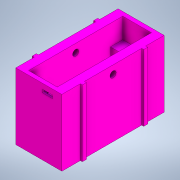
# Autodesk Inventor part: hull_servo
Saved by Autodesk Inventor 2020 (Build 240168000, 168)
## iProperties
Created: 2019-09-18
Part Number: hull_servo
Material: Generic
Document SubType Name: Modeling
Designer: suchanek
Density: 1 g/cm^3
Appearance: Default
Author: suchanek
Autodesk Inventor part; units mm, degrees
ref_plane "YZ Plane" through (0, 0, 0) normal (1, 0, 0) x (0, 1, 0)
ref_plane "XZ Plane" through (0, 0, 0) normal (0, 1, 0) x (-1, 0, 0)
ref_plane "XY Plane" through (0, 0, 0) normal (0, 0, 1) x (1, 0, 0)
sketch "Sketch1" plane through (0, 0, 0) normal (0, 1, 0) x (-1, 0, 0)
  line L0 (-14, 34) -> (14, 34)
  line L1 (14, 34) -> (14, -34)
  line L2 (14, -34) -> (-14, -34)
  line L3 (-14, -34) -> (-14, 34)
  line L4 (-14, 34) -> (14, -34) construction
  line L5 (14, 34) -> (-14, -34) construction
  line L6 (-22.5, 50) -> (22.5, 50)
  line L7 (22.5, 50) -> (22.5, -50)
  line L8 (22.5, -50) -> (-22.5, -50)
  line L9 (-22.5, -50) -> (-22.5, 50)
  line L10 (-22.5, 50) -> (22.5, -50) construction
  line L11 (22.5, 50) -> (-22.5, -50) construction
  line L12 (22.5, -28) -> (24.5, -28)
  line L13 (24.5, -28) -> (24.5, -32)
  line L14 (24.5, -32) -> (22.5, -32)
  line L15 (22.5, -32) -> (22.5, -28)
  line L16 (0, 0) -> (0, -11.0909)
  line L17 (0, -11.0909) -> (0, 0)
  line L18 (0, 0) -> (9.2257, 0)
  line L19 (22.5, 28) -> (24.5, 28)
  line L20 (24.5, 28) -> (24.5, 32)
  line L21 (24.5, 32) -> (22.5, 32)
  line L22 (22.5, 32) -> (22.5, 28)
  line L23 (-22.5, -28) -> (-24.5, -28)
  line L24 (-24.5, -28) -> (-24.5, -32)
  line L25 (-24.5, -32) -> (-22.5, -32)
  line L26 (-22.5, -32) -> (-22.5, -28)
  line L27 (-22.5, 28) -> (-24.5, 28)
  line L28 (-22.5, 32) -> (-22.5, 28)
  line L29 (-24.5, 32) -> (-22.5, 32)
  line L30 (-24.5, 28) -> (-24.5, 32)
  dimension "d0" = 28
  dimension "d1" = 68
  dimension "d2" = 45
  dimension "d3" = 100
  dimension "d11" = 2
  dimension "d12" = 4
  dimension "d13" = 28
  constraints: 62 end point, 12 symmetric about line, 7 equal length, 4 horizontal, 4 midpoint, 3 perpendicular, 1 point on line, 1 vertical
  measures "d0" distance of L1.end L2.end
  measures "d1" distance of L0.end L1.end
  measures "d2" distance of L7.end L8.end
  measures "d3" distance of L6.end L7.end
  measures "d11" distance of L13.end L14.end
  measures "d12" distance of L12.end L13.end
  measures "d13" distance from line of L16.start L12
extrude "Extrusion1" add sketch "Sketch1" against normal blind 10 contours L0 L1 L2 L3 | L6 L7 L8 L9 | L9 L27 L30 L29 | L21 L20 L19 L7 | L9 L25 L24 L23 | L12 L13 L14 L7
extrude "Extrusion2" add sketch "Sketch1" along normal blind 55
sketch "Sketch2" plane through (0, 55, 0) normal (0, 1, 0) x (1, 0, 0)
  line L0 (-14, -46) -> (14, -46)
  line L1 (14, -46) -> (14, 46)
  line L2 (14, 46) -> (-14, 46)
  line L3 (-14, 46) -> (-14, -46)
  line L4 (-14, -46) -> (14, 46) construction
  line L5 (14, -46) -> (-14, 46) construction
  line L6 (-14, 34) -> (-14, -34) projected
  line L7 (-14, -34) -> (14, -34) projected
  line L8 (14, -34) -> (14, 34) projected
  line L9 (14, 34) -> (-14, 34) projected
  point P0 (0, 0)
  dimension "d8" = 12
  constraints: 12 end point, 2 midpoint, 2 parallel, 1 collinear, 1 horizontal, 1 perpendicular
  measures "d8" distance between parallel lines of L0 L7
extrude "Extrusion3" cut sketch "Sketch2" against normal blind 20 contours L3 L7 L1 L0 | L3 L2 L1 L9
sketch "Sketch3" plane through (22.5, -10, 28) normal (1, 0, 0) x (0, 0, -1)
  line L0 (0, 0) -> (0, 65) projected
  line L1 (0, 65) -> (56, 65) projected
  line L2 (56, 0) -> (56, 65) projected
  circle A0 centre (28, 57) radius 3
  point P0 (28, 10)
  dimension "d18" = 6
  dimension "d19" = 8
  constraints: 1 centre point, 1 vertical alignment
  measures "d18" diameter of A0
  measures "d19" distance from line of L1 A0.centre
extrude "Extrusion4" cut sketch "Sketch3" against normal through all
sketch "Sketch6" plane through (14, 0, 34) normal (0, 0, -1) x (-1, 0, 0)
  line L0 (28, 0) -> (0, 0) projected
  line L1 (28, 35) -> (0, 35) projected
  line L2 (11.5, 0) -> (16.5, 0)
  line L3 (16.5, 0) -> (16.5, 35)
  line L4 (16.5, 35) -> (11.5, 35)
  line L5 (11.5, 35) -> (11.5, 0)
  line L6 (14, 0) -> (14, 3.571)
  dimension "d23" = 5
  constraints: 10 end point, 2 parallel, 2 point on line, 1 horizontal, 1 perpendicular, 1 vertical, 1 other
  measures "d23" distance between parallel lines of L3 L5
extrude "Extrusion6" cut sketch "Sketch6" against normal blind 3
sketch "Sketch7" plane through (0, 35, 0) normal (0, 1, 0) x (1, 0, 0)
  line L0 (2.5, -37) -> (-2.5, -37) projected
  line L1 (14, -46) -> (-14, -46) projected
  line L2 (-2.5, -37) -> (2.5, -37)
  line L3 (2.5, -37) -> (2.5, -46)
  line L4 (2.5, -46) -> (-2.5, -46)
  line L5 (-2.5, -46) -> (-2.5, -37)
  line L6 (2.5, -34) -> (2.5, -37) projected
  point P0 (0, 0)
  constraints: 8 end point, 2 parallel, 1 collinear, 1 horizontal, 1 perpendicular, 1 point on line
extrude "Extrusion7" cut sketch "Sketch7" against normal blind 4
sketch "Sketch8" plane through (14, 55, 46) normal (0, 0, -1) x (-1, 0, 0)
  line L0 (16.5, -20) -> (16.5, -24) projected
  line L1 (16.5, -24) -> (11.5, -24)
  line L2 (11.5, -24) -> (3, -8)
  line L3 (3, -8) -> (8, -8)
  line L4 (8, -8) -> (16.5, -24)
  line L5 (11.5, -55) -> (11.5, -20) projected
  line L6 (10.5, -8) -> (0.5, -8)
  line L7 (0.5, -8) -> (0.5, -5)
  line L8 (0.5, -5) -> (10.5, -5)
  line L9 (10.5, -5) -> (10.5, -8)
  line L10 (14, -24) -> (14, -20)
  line L11 (0, 0) -> (28, 0) projected
  line L12 (5.5, -8) -> (5.5, -9.1471)
  point P0 (14, -55)
  point P1 (-8.5, 0)
  dimension "d28" = 3
  dimension "d29" = 10
  dimension "d30" = 5
  dimension "d36" = 9
  constraints: 20 end point, 4 parallel, 2 horizontal, 2 midpoint, 2 vertical, 1 collinear, 1 perpendicular, 1 point on line, 1 symmetric about line, 1 other
  measures "d28" distance of L8.end L6.start
  measures "d29" distance of L7.end L8.end
  measures "d30" distance between parallel lines of L11 L8
  measures "d36" distance from line of point (-8.5, 0) L7
extrude "Extrusion8" cut sketch "Sketch8" against normal blind 2 contours L1 L2 L3 L4
extrude "Extrusion9" cut sketch "Sketch8" against normal through all contours L3 L6 L7 L8 L9
body "Solid1"
